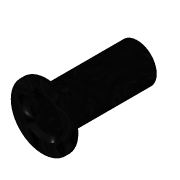
# Autodesk Inventor part: 50_ETL_Motionpart1_v0
Saved by Autodesk Inventor 2022 (Build 260153000, 153)
## iProperties
Created: 2021-12-31
Part Number: 50_ETL_Motionpart1_v0
Material: Generisch
Document SubType Name: Modeling
Designer: diederichbenedict
Density: 1 g/cm^3
Appearance: Schwarz
Author: diederichbenedict
Autodesk Inventor part; units mm, degrees
ref_plane "YZ Plane" through (0, 0, 0) normal (1, 0, 0) x (0, 1, 0)
ref_plane "XZ Plane" through (0, 0, 0) normal (0, 1, 0) x (-1, 0, 0)
sketch "Skizze1" plane through (0, 0, 0) normal (0, 0, 1) x (1, 0, 0)
  arc A0 (-2.8009, 5.3061) -> (2.8009, 5.3061) centre (0, 0) ccw projected
  circle A1 centre (0, 0) radius 5 projected
  circle A2 centre (0, 0) radius 4.9
  circle A3 centre (0, 0) radius 4.05
  point P0 (0, 0)
  dimension "d0" = 0.1
  dimension "d1" = 8.1
  constraints: 2 centre point, 1 coincident
  measures "d0" radial gap between concentric circles of A1 A2
  measures "d1" diameter of A3
extrude "Extrusion1" add sketch "Skizze1" along normal blind 6 and the other way blind 18 contours A2
sketch "Skizze2" plane through (0, 0, 6) normal (0, 0, 1) x (1, 0, 0)
  circle A0 centre (0, 0) radius 4.9 projected
  circle A1 centre (0, 0) radius 8.5508 projected
  circle A2 centre (0, 0) radius 7.7 projected
  circle A3 centre (0, 0) radius 8.0508
  point P0 (0, 0)
  dimension "d4" = 0.5
  constraints: 1 centre point
  measures "d4" radial gap between concentric circles of A1 A3
extrude "Extrusion2" add sketch "Skizze2" against normal blind 1 contours A2 | A3
chamfer "Fase1" distance 1 angle 45 2 edges at (-4.9, 0, 5) (-4.05, 0, 6)
sketch "Skizze3" plane through (0, 0, 5) normal (0, 0, -1) x (-1, 0, 0)
  circle A0 centre (0, 0) radius 4.9 projected
  circle A1 centre (0, 0) radius 5.05 projected
  circle A2 centre (0, 0) radius 4.1058
  circle A3 centre (0, 0) radius 6.4267
  point P0 (0, 0)
  constraints: 2 centre point, 2 coincident
ref_plane "Arbeitsebene1" through (-19.3, -19.3, 3.2) normal (0, 0, 1) x (1, 0, 0)
extrude "Extrusion3" add sketch "Skizze3" along normal up to surface (1.8 mm away)
